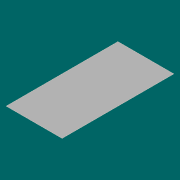
# Autodesk Inventor part: A1-18002-100-01 Floor
Saved by Autodesk Inventor 2017 (Build 210142000, 142)
## iProperties
Created: 2018-01-23
Part Number: A1-18002-100-01 Floor
Material: Steel, Mild
Document SubType Name: Modeling
Designer: Graeme_Van_Dongen
Density: 7.85 g/cm^3
Appearance: Steel
Mass: 70894.8 g
Surface Area: 59680.2 cm^2
Volume: 9031.19 cm^3
Description: 96" x 48" x 11Ga SHEET, A569
Author: Graeme_Van_Dongen
Autodesk Inventor part; units mm, degrees
ref_plane "YZ Plane" through (0, 0, 0) normal (1, 0, 0) x (0, 1, 0)
ref_plane "XZ Plane" through (0, 0, 0) normal (0, 1, 0) x (-1, 0, 0)
ref_plane "XY Plane" through (0, 0, 0) normal (0, 0, 1) x (1, 0, 0)
sketch "Sketch1" plane through (0, 0, 0) normal (0, 1, 0) x (-1, 0, 0)
  line L0 (609.6, 1219.2) -> (-609.6, 1219.2)
  line L1 (-609.6, 1219.2) -> (-609.6, -1219.2)
  line L2 (-609.6, -1219.2) -> (609.6, -1219.2)
  line L3 (609.6, -1219.2) -> (609.6, 1219.2)
  line L4 (609.6, 1219.2) -> (-609.6, -1219.2) construction
  line L5 (-609.6, 1219.2) -> (609.6, -1219.2) construction
  point P0 (0, 0)
  dimension "d0" = 1219.2
  dimension "d1" = 2438.4
  constraints: 12 end point, 2 midpoint, 2 parallel, 1 horizontal, 1 perpendicular
  measures "d0" distance of L2.end L1.end
  measures "d1" distance of L1.end L0.end
extrude "Extrusion1" add sketch "Sketch1" along normal blind 3.0378
body "Solid1"
